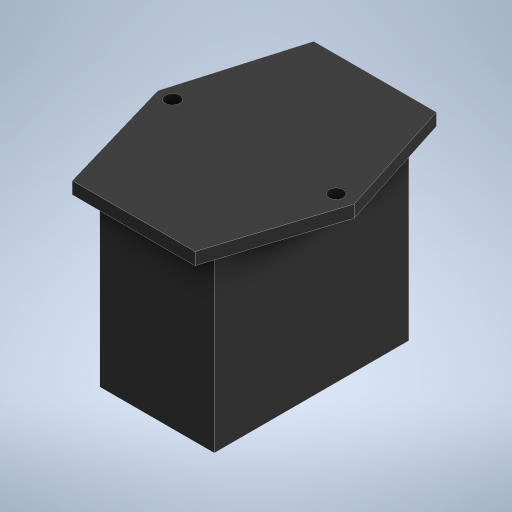
# Autodesk Inventor part: Kaltstecker
Saved by Autodesk Inventor 2024 (Build 280153000, 153)
## iProperties
Created: 2026-05-31
Part Number: Kaltstecker
Material: Gummi, Silikon
Document SubType Name: Modeling
Designer: maxim
Density: 1.25 g/cm^3
Appearance: Gummi - Schwarz
Author: maxim
Autodesk Inventor part; units mm, degrees
ref_plane "YZ Plane" through (0, 0, 0) normal (1, 0, 0) x (0, 1, 0)
ref_plane "XZ Plane" through (0, 0, 0) normal (0, 1, 0) x (-1, 0, 0)
ref_plane "XY Plane" through (0, 0, 0) normal (0, 0, 1) x (1, 0, 0)
sketch "Skizze1" plane through (0, 0, 0) normal (0, 0, 1) x (1, 0, 0)
  line L0 (-14, -23.8) -> (-14, 23.8)
  line L1 (-14, 23.8) -> (14, 23.8)
  line L2 (14, 23.8) -> (14, -23.8)
  line L3 (14, -23.8) -> (-14, -23.8)
  line L4 (-14, -23.8) -> (14, 23.8) construction
  line L5 (-14, 23.8) -> (14, -23.8) construction
  point P0 (0, 0)
  dimension "d0" = 47.6
  dimension "d1" = 28
  constraints: 12 end point, 2 midpoint, 2 parallel, 1 perpendicular, 1 vertical
  measures "d0" distance of L0.start L0.end
  measures "d1" distance of L0.end L1.end
extrude "Extrusion1" add sketch "Skizze1" against normal blind 43
sketch "Skizze2" plane through (0, 0, 0) normal (0, 0, 1) x (1, 0, 0)
  line L0 (15, -29.5) -> (-15, -29.5)
  line L1 (-15, 29.5) -> (15, 29.5)
  line L2 (14, 23.8) -> (-14, 23.8) projected
  line L3 (-15, 29.5) -> (-23.5996, 0)
  line L4 (-23.5996, 0) -> (-15, -29.5)
  line L5 (15, -29.5) -> (24.4004, 0)
  line L6 (24.4004, 0) -> (15, 29.5)
  point P0 (0, 0)
  point P1 (0, 0)
  dimension "d4" = 5.7
  dimension "d15" = 59
  dimension "d16" = 48
  dimension "d17" = 30
  constraints: 12 end point, 2 horizontal alignment, 1 coincident, 3 other
  measures "d4" distance between parallel lines of L2 L1
  measures "d15" distance between parallel lines of L0 L1
  measures "d16" distance of L5.end L3.end
  measures "d17" distance of L1.start L1.end
extrude "Extrusion2" add sketch "Skizze2" along normal blind 3
sketch "Skizze3" plane through (0, 0, 3) normal (0, 0, 1) x (1, 0, 0)
  line L0 (15, 29.5) -> (-15, 29.5) projected
  line L1 (0, 29.5) -> (0, -29.5)
  line L2 (-15, -29.5) -> (15, -29.5) projected
  point P0 (0, 0)
  point P1 (-20, 0)
  point P2 (20, 0)
  dimension "d7" = 40
  constraints: 2 end point, 2 midpoint, 1 symmetric about line
  measures "d7" diameter of point (-20, 0) L1
hole "Bohrung1" at (-20, 0, 3) at (20, 0, 3) direction (0, 0, -1) diameter 3.5 end through all
